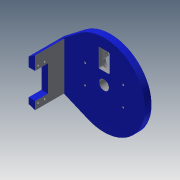
# Autodesk Inventor part: otocni_kruh(svrchni)
Saved by Autodesk Inventor 2013 (Build 170138000, 138)
## iProperties
Created: 2013-05-25
Part Number: otocni_kruh(svrchni)
Material: Generic
Document SubType Name: Modeling
Designer: idle-rug
Density: 1 g/cm^3
Author: idle-rug
Autodesk Inventor part; units mm, degrees
ref_plane "YZ Plane" through (0, 0, 0) normal (1, 0, 0) x (0, 1, 0)
ref_plane "XZ Plane" through (0, 0, 0) normal (0, 1, 0) x (-1, 0, 0)
ref_plane "XY Plane" through (0, 0, 0) normal (0, 0, 1) x (1, 0, 0)
sketch "Sketch1" plane through (0, 0, 0) normal (0, 1, 0) x (-1, 0, 0)
  circle A0 centre (0, 0) radius 60
  circle A1 centre (0, 0) radius 3
  dimension "d0" = 120
  dimension "d1" = 6
  constraints: 2 centre point, 2 coincident
  measures "d0" diameter of A0
  measures "d1" diameter of A1
extrude "Extrusion1" add sketch "Sketch1" along normal blind 10
sketch "Sketch2" plane through (0, 0, 0) normal (0, -1, 0) x (1, 0, 0)
  circle A0 centre (0, 0) radius 60 projected
  line L0 (0, 0) -> (24.3, 0)
  line L1 (24.3, 0) -> (29.3, 0)
  line L2 (0, 0) -> (-24.3, 0)
  line L3 (-24.3, 0) -> (-29.3, 0)
  line L4 (-24.3, 30) -> (-34.3, 30)
  line L5 (-34.3, 30) -> (-34.3, -30)
  line L6 (-34.3, -30) -> (-24.3, -30)
  line L7 (-24.3, -30) -> (-24.3, 30)
  line L8 (-24.3, 30) -> (-34.3, -30) construction
  line L9 (-34.3, 30) -> (-24.3, -30) construction
  line L10 (34.3, 30) -> (24.3, 30)
  line L11 (24.3, 30) -> (24.3, -30)
  line L12 (24.3, -30) -> (34.3, -30)
  line L13 (34.3, -30) -> (34.3, 30)
  line L14 (34.3, 30) -> (24.3, -30) construction
  line L15 (24.3, 30) -> (34.3, -30) construction
  line L16 (-29.3, 0) -> (-29.3, 15)
  line L17 (-29.3, 0) -> (-29.3, -15)
  line L18 (29.3, 0) -> (29.3, 15)
  line L19 (29.3, 0) -> (29.3, -15)
  circle A1 centre (29.3, -15) radius 1.5
  circle A2 centre (29.3, 15) radius 1.5
  circle A3 centre (-29.3, 15) radius 1.5
  circle A4 centre (-29.3, -15) radius 1.5
  dimension "d4" = 24.3
  dimension "d5" = 5
  dimension "d6" = 24.3
  dimension "d7" = 5
  dimension "d8" = 10
  dimension "d9" = 60
  dimension "d10" = 60
  dimension "d11" = 15
  dimension "d12" = 15
  dimension "d13" = 15
  dimension "d14" = 15
  dimension "d15" = 3
  dimension "d16" = 3
  dimension "d17" = 3
  dimension "d18" = 3
  constraints: 40 end point, 6 parallel, 5 collinear, 4 centre point, 4 coincident, 4 midpoint, 3 horizontal, 2 perpendicular
  measures "d4" distance of L0.start L0.end
  measures "d5" distance of L0.end L1.end
  measures "d6" distance of L0.start L2.end
  measures "d7" distance of L2.end L3.end
  measures "d8" distance of L6.end L5.end
  measures "d9" distance of L5.end L4.end
  measures "d10" distance of L11.end L10.end
  measures "d11" distance of L3.end L16.end
  measures "d12" distance of L3.end L17.end
  measures "d13" distance of L1.end L18.end
  measures "d14" distance of L1.end L19.end
  measures "d15" diameter of A1
  measures "d16" diameter of A2
  measures "d17" diameter of A3
  measures "d18" diameter of A4
extrude "Extrusion2" cut sketch "Sketch2" against normal blind 10 contours A1 | A2 | A3 | A4
sketch "Sketch3" plane through (0, 0, 0) normal (0, -1, 0) x (1, 0, 0)
  circle A0 centre (0, 0) radius 60 projected
  line L0 (0, 0) -> (-71.2, 0)
  line L1 (-71.2, 0) -> (-71.2, -34.25)
  line L2 (-71.2, -34.25) -> (-71.2, 20.75)
  line L3 (-24.1381, -54.9304) -> (-71.2, -34.25)
  line L4 (-36.7367, 47.4386) -> (-71.2, 20.75)
  arc A1 (-36.7367, 47.4386) -> (-24.1381, -54.9304) centre (0, 0) ccw
  dimension "d31" = 71.2
  dimension "d32" = 34.25
  dimension "d33" = 55
  constraints: 10 end point, 4 point on circle, 2 tangent, 1 centre point, 1 concentric, 1 horizontal, 1 perpendicular, 1 point on line
  measures "d31" distance of L0.start L0.end
  measures "d32" distance of L0.end L1.end
  measures "d33" distance of L1.end L2.end
extrude "Extrusion3" add sketch "Sketch3" against normal blind 10 contours A0 L0 L2 L4 | L3 L1 L0 A0
sketch "Sketch4" plane through (0, 0, 0) normal (0, -1, 0) x (1, 0, 0)
  line L0 (-61.2, 20.75) -> (-61.2, -34.25)
  line L1 (-71.2, -34.25) -> (-71.2, 20.75)
  line L2 (-61.2, 28.494) -> (-61.2, -38.6443)
  line L3 (-61.2, -38.6443) -> (-71.2, -34.25)
  line L4 (-71.2, -34.25) -> (-71.2, 20.75)
  line L5 (-71.2, -34.25) -> (-71.2, 20.75) projected
  line L6 (-61.2, 28.494) -> (-71.2, 20.75)
  dimension "d36" = 10
  constraints: 12 end point, 2 parallel, 1 collinear
  measures "d36" distance of L0.end L1.start
extrude "Extrusion4" add sketch "Sketch4" along normal blind 43
sketch "Sketch6" plane through (0, -43, 0) normal (0, -1, 0) x (1, 0, 0)
  line L0 (-71.2, 20.75) -> (-71.2, -34.25) projected
  line L1 (-71.2, -34.25) -> (-61.2, -38.6443) projected
  line L2 (-61.2, -38.6443) -> (-61.2, 28.494) projected
  line L3 (-61.2, 28.494) -> (-71.2, 20.75) projected
  point P0 (0, 0)
extrude "Extrusion5" add sketch "Sketch6" along normal blind 5
sketch "Sketch7" plane through (0, 10, 0) normal (0, 1, 0) x (1, 0, 0)
  arc A0 (-36.7367, -47.4386) -> (-24.1381, 54.9304) centre (0, 0) ccw projected
  line L0 (-24.1381, 54.9304) -> (-71.2, 34.25) projected
  line L1 (-71.2, 34.25) -> (-71.2, -20.75) projected
  line L2 (-71.2, -20.75) -> (-36.7367, -47.4386) projected
  line L3 (-71.2, 34.25) -> (-71.2, -20.75)
  line L4 (-71.2, -20.75) -> (-71.2, -24.75)
  line L5 (-71.2, 34.25) -> (-71.2, 38.25)
  line L6 (-71.2, 38.25) -> (-20.2127, 56.4929)
  line L7 (-71.2, -24.75) -> (-36.7367, -47.4386)
  line L8 (-71.2, -20.75) -> (-36.7367, -47.4386)
  line L9 (-71.2, 34.25) -> (-24.1381, 54.9304)
  arc A1 (-36.7367, -47.4386) -> (-24.1381, 54.9304) centre (0, 0) ccw projected
  arc A2 (-20.2127, 56.4929) -> (-24.1381, 54.9304) centre (0, 0) ccw
  dimension "d45" = 4
  dimension "d46" = 4
  constraints: 14 end point, 5 point on circle, 4 collinear, 2 point on line, 2 tangent, 1 centre point
  measures "d45" distance of L1.end L4.end
  measures "d46" distance of L0.end L5.end
extrude "Extrusion6" add sketch "Sketch7" against normal blind 10 contours L7 L4 L2 | A0 L0 L5 L6
sketch "Sketch8" plane through (0, 0, 0) normal (0, -1, 0) x (1, 0, 0)
  line L0 (-71.2, -38.25) -> (-20.2127, -56.4929) projected
  line L1 (-36.7367, 47.4386) -> (-71.2, 24.75) projected
  line L2 (-71.2, 24.75) -> (-71.2, 20.75) projected
  line L3 (-61.2, 28.494) -> (-71.2, 20.75) projected
  line L4 (-61.2, 28.494) -> (-61.2, 31.3334)
  line L5 (-61.2, -38.6443) -> (-61.2, -41.8279)
  line L6 (-71.2, -34.25) -> (-71.2, -38.25)
  line L7 (-71.2, -38.25) -> (-61.2, -41.8279)
  line L8 (-71.2, -34.25) -> (-61.2, -38.6443)
  line L9 (-71.2, -34.25) -> (-61.2, -38.6443) projected
  line L10 (-71.2, 20.75) -> (-71.2, 24.75)
  line L11 (-71.2, 24.75) -> (-61.2, 31.3334)
  line L12 (-61.2, 28.494) -> (-71.2, 20.75)
  constraints: 16 end point, 6 collinear, 2 parallel, 1 point on line
extrude "Extrusion7" add sketch "Sketch8" along normal blind 48
sketch "Sketch9" plane through (-71.2, -48, -38.25) normal (-1, 0, 0) x (0, 0, 1)
  line L0 (63, 58) -> (63, 0) projected
  line L1 (38.25, 48) -> (38.25, 13)
  line L2 (38.25, 13) -> (4, 13)
  line L3 (4, 13) -> (53.7, 13)
  line L4 (48.95, 23) -> (8.75, 23)
  line L5 (8.75, 23) -> (8.75, 3)
  line L6 (8.75, 3) -> (48.95, 3)
  line L7 (48.95, 3) -> (48.95, 23)
  line L8 (48.95, 23) -> (8.75, 3) construction
  line L9 (8.75, 23) -> (48.95, 3) construction
  circle A0 centre (53.7, 17.95) radius 1.5
  circle A1 centre (53.7, 8.05) radius 1.5
  circle A2 centre (4, 17.95) radius 1.5
  circle A3 centre (4, 8.05) radius 1.5
  point P0 (28.85, 13)
  dimension "d51" = 35
  dimension "d54" = 34.25
  dimension "d55" = 49.7
  dimension "d56" = 40.2
  dimension "d60" = 3
  dimension "d61" = 3
  dimension "d62" = 3
  dimension "d63" = 3
  constraints: 18 end point, 4 centre point, 3 midpoint, 3 parallel, 2 perpendicular, 1 horizontal, 1 point on line
  measures "d51" distance of L1.start L1.end
  measures "d54" distance of L1.end L2.end
  measures "d55" distance of L2.end L3.end
  measures "d56" distance of L6.end L5.end
  measures "d60" diameter of A0
  measures "d61" diameter of A1
  measures "d62" diameter of A2
  measures "d63" diameter of A3
extrude "Extrusion8" cut sketch "Sketch9" against normal blind 10
sketch "Sketch10" plane through (0, -48, 0) normal (0, -1, 0) x (1, 0, 0)
  line L0 (-71.2, 24.75) -> (-71.2, -38.25) projected
  line L1 (-71.2, -38.25) -> (-61.2, -41.8279) projected
  line L2 (-61.2, -41.8279) -> (-61.2, 31.3334) projected
  line L3 (-61.2, 31.3334) -> (-71.2, 24.75) projected
  point P0 (0, 0)
extrude "Extrusion9" cut sketch "Sketch10" against normal blind 3
sketch "Sketch11" plane through (0, 10, 0) normal (0, 1, 0) x (1, 0, 0)
  circle A0 centre (0, -37.2) radius 7.1045
  circle A1 centre (0, -37.2) radius 2
  dimension "d70" = 14.209
  dimension "d71" = 4
  constraints: 2 centre point, 1 coincident
  measures "d70" diameter of A0
  measures "d71" diameter of A1
extrude "Extrusion10" cut sketch "Sketch11" against normal blind 10 contours A1
sketch "Sketch12" plane through (0, 10, 0) normal (0, 1, 0) x (1, 0, 0)
  circle A0 centre (0, -37.2) radius 2 projected
  circle A1 centre (0, -37.2) radius 4
  dimension "d74" = 8
  constraints: 1 centre point, 1 coincident
  measures "d74" diameter of A1
extrude "Extrusion11" cut sketch "Sketch12" against normal blind 10
sketch "Sketch13" plane through (0, 0, 0) normal (0, -1, 0) x (1, 0, 0)
  circle A0 centre (0, 37.2) radius 4 projected
  circle A1 centre (0, 37.2) radius 4 projected
  circle A2 centre (0, 37.2) radius 7.5
  line L0 (0, 29.7) -> (0, 19.7)
  line L1 (0, 19.7) -> (-24.3, 19.7)
  line L2 (-24.3, 19.7) -> (-24.3, 54.859)
  line L3 (0, 19.7) -> (24.3, 19.7)
  line L4 (24.3, 19.7) -> (24.3, 54.859)
  arc A3 (24.3, 54.859) -> (-24.3, 54.859) centre (0, 0) ccw
  dimension "d78" = 15
  dimension "d79" = 10
  constraints: 10 end point, 2 perpendicular, 2 point on circle, 1 centre point, 1 coincident, 1 vertical alignment, 2 other
  measures "d79" distance of L0.start L0.end
extrude "Extrusion12" cut sketch "Sketch13" against normal blind 6 contours A2 | L1 L2 A3 L4 L3
sketch "Sketch14" plane through (0, 6, 0) normal (0, -1, 0) x (1, 0, 0)
  line L0 (-24.3, 19.7) -> (-24.3, 54.859) projected
  line L1 (24.3, 19.7) -> (-24.3, 19.7) projected
  line L2 (24.3, 54.859) -> (24.3, 19.7) projected
  arc A0 (24.3, 54.859) -> (-24.3, 54.859) centre (0, 0) ccw projected
  line L3 (-24.3, 19.7) -> (-10, 19.7)
  line L4 (-10, 19.7) -> (-10, 54.859)
  line L5 (-10, 54.859) -> (-24.3, 54.859)
  line L6 (-24.3, 54.859) -> (-24.3, 19.7)
  line L7 (24.3, 19.7) -> (10, 19.7)
  line L8 (10, 19.7) -> (10, 54.859)
  line L9 (10, 54.859) -> (24.3, 54.859)
  line L10 (24.3, 54.859) -> (24.3, 19.7)
  line L11 (-24.3, 54.859) -> (24.3, 54.859)
  dimension "d82" = 14.3
  dimension "d83" = 14.3
  constraints: 18 end point, 4 parallel, 2 horizontal, 2 perpendicular, 1 collinear
  measures "d82" distance of L5.end L4.end
  measures "d83" distance of L8.end L9.end
extrude "Extrusion13" add sketch "Sketch14" along normal blind 6 contours L0 L5 L4 L1 | A0 L9 L11 L5 | L2 L1 L8 L9
sketch "Sketch16" plane through (0, 0, 0) normal (0, -1, 0) x (1, 0, 0)
  line L0 (-10, 19.7) -> (-10, 29.7) projected
  line L1 (-10, 19.7) -> (-10, 54.859) projected
  line L2 (-10, 44.859) -> (-10, 54.859) projected
  line L3 (10, 54.859) -> (10, 44.859) projected
  line L4 (10, 54.859) -> (10, 19.7) projected
  line L5 (10, 29.7) -> (10, 19.7) projected
  arc A0 (-20.2127, -56.4929) -> (-36.7367, 47.4386) centre (0, 0) ccw projected
  circle A1 centre (0, 0) radius 3 projected
  circle A2 centre (0, 0) radius 24.3
  line L6 (-10, 54.859) -> (-24.3, 54.859)
  line L7 (-24.3, 54.859) -> (-24.3, 19.859)
  line L8 (-24.3, 19.859) -> (-10, 19.7)
  line L9 (10, 54.859) -> (24.3, 54.859)
  line L10 (24.3, 54.859) -> (24.3, 19.859)
  line L11 (24.3, 19.859) -> (10, 19.7)
  dimension "d90" = 48.6
  dimension "d91" = 14.3
  dimension "d92" = 35
  dimension "d93" = 14.3
  dimension "d94" = 35
  constraints: 12 end point, 2 perpendicular, 2 point on circle, 1 centre point, 1 coincident
  measures "d90" diameter of A2
  measures "d91" distance of L1.end L6.end
  measures "d92" distance of L6.end L7.end
  measures "d93" distance of L3.start L9.end
  measures "d94" distance of L9.end L10.end
extrude "Extrusion15" add sketch "Sketch16" along normal blind 24 contours L8 A2 L0 | A2 L8 L7 L6 L1 L0 | A2 L11 L4 | L4 L3 L9 L10 L11 A2
sketch "Sketch17" plane through (24.3, 0, 54.859) normal (1, 0, 0) x (0, 0, -1)
  line L0 (0, 0) -> (35, 0) projected
  line L1 (0, 0) -> (0, -24) projected
  line L2 (0, -24) -> (19.125, -24)
  line L3 (0, 0) -> (4.589, 0)
  line L4 (4.589, 0) -> (19.125, -24)
  line L5 (0, 0) -> (0, -24)
  point P0 (54.859, 0)
  dimension "d97" = 19.125
  dimension "d98" = 4.589
  constraints: 8 end point, 1 perpendicular, 1 point on line
  measures "d97" distance of L1.end L2.end
  measures "d98" distance of L0.start L3.end
extrude "Extrusion16" add sketch "Sketch17" along normal blind 10
sketch "Sketch18" plane through (-24.3, 0, 19.859) normal (-1, 0, 0) x (0, 0, 1)
  line L0 (0, 0) -> (35, 0) projected
  line L1 (35, 0) -> (35, -24) projected
  line L2 (35, -24) -> (15.875, -24)
  line L3 (35, -24) -> (-0.159, -24) projected
  line L4 (35, 0) -> (30.411, 0)
  line L5 (30.411, 0) -> (15.875, -24)
  point P0 (-19.859, 0)
  point P1 (25, -24)
  point P2 (9.841, -24)
  dimension "d101" = 19.125
  dimension "d102" = 4.589
  constraints: 6 end point, 2 point on line
  measures "d101" distance of L1.end L2.end
  measures "d102" distance of L0.end L4.end
extrude "Extrusion17" add sketch "Sketch18" along normal blind 10
sketch "Sketch23" plane through (0, 10, 0) normal (0, 1, 0) x (1, 0, 0)
  circle A0 centre (0, 0) radius 3 projected
  arc A1 (-36.7367, -47.4386) -> (-20.2127, 56.4929) centre (0, 0) ccw projected
  circle A2 centre (0, 0) radius 7.5
  dimension "d123" = 15
  constraints: 1 centre point, 1 coincident
  measures "d123" diameter of A2
extrude "Extrusion22" cut sketch "Sketch23" against normal blind 10
sketch "Sketch24" plane through (0, 0, 0) normal (0, -1, 0) x (1, 0, 0)
  arc A0 (-20.2127, -56.4929) -> (-36.7367, 47.4386) centre (0, 0) ccw projected
  circle A1 centre (0, 0) radius 17.5
  dimension "d126" = 35
  constraints: 1 centre point, 1 coincident
  measures "d126" diameter of A1
extrude "Extrusion23" add sketch "Sketch24" along normal blind 2
sketch "Sketch26" plane through (0, -2, 0) normal (0, -1, 0) x (1, 0, 0)
  circle A0 centre (0, 0) radius 17.5 projected
  circle A1 centre (0, 0) radius 5
  dimension "d131" = 10
  constraints: 1 centre point, 1 coincident
  measures "d131" diameter of A1
extrude "Extrusion24" cut sketch "Sketch26" against normal blind 2 contours A1
sketch "Sketch30" plane through (0, 10, 0) normal (0, 1, 0) x (1, 0, 0)
  arc A0 (-36.7367, -47.4386) -> (-20.2127, 56.4929) centre (0, 0) ccw projected
  line L0 (-20.2127, 56.4929) -> (-71.2, 38.25) projected
  line L1 (-71.2, 38.25) -> (-71.2, -24.75) projected
  line L2 (-71.2, -24.75) -> (-36.7367, -47.4386) projected
  line L3 (-71.2, 38.25) -> (-24.5824, 58.0061)
  line L4 (-71.2, -24.75) -> (-38.3769, -49.9621)
  line L5 (-71.2, 38.25) -> (-71.2, -24.75)
  line L6 (-71.2, 38.25) -> (-20.2127, 56.4929)
  line L7 (-71.2, -24.75) -> (-36.7367, -47.4386)
  arc A1 (-36.7367, -47.4386) -> (-20.2127, 56.4929) centre (0, 0) ccw
  arc A2 (-38.3769, -49.9621) -> (-24.5824, 58.0061) centre (0, 0) ccw
  dimension "d141" = 63
  constraints: 10 end point, 4 point on circle, 3 collinear, 2 centre point, 2 tangent, 1 concentric
  measures "d141" radius of A2
extrude "Extrusion27" add sketch "Sketch30" against normal blind 10 contours A0 L0 L3 A2 L4 L2
sketch "Sketch31" plane through (0, 10, 0) normal (0, 1, 0) x (1, 0, 0)
  circle A0 centre (0, -37.2) radius 4 projected
  line L0 (-71.2, 38.25) -> (-71.2, -24.75) projected
  line L1 (0, -33.2) -> (0, -25.7)
  circle A1 centre (0, -25.7) radius 7.5
  dimension "d144" = 7.5
  constraints: 2 end point, 2 vertical alignment, 1 coincident, 1 parallel, 3 other
  measures "d144" distance of L1.start L1.end
extrude "Extrusion28" cut sketch "Sketch31" against normal blind 10 contours A1
sketch "Sketch32" plane through (0, 10, 0) normal (0, 1, 0) x (1, 0, 0)
  line L0 (-71.2, 38.25) -> (-71.2, -24.75) projected
  circle A0 centre (0, -37.2) radius 4 projected
  circle A1 centre (0, -25.7) radius 7.5 projected
  line L1 (0, -33.2) -> (-3, -33.2)
  arc A2 (0, -33.2) -> (4.5, -19.7) centre (0, -25.7) ccw projected
  line L2 (-3, -33.2) -> (3, -33.2)
  line L3 (3, -32.2) -> (-3, -32.2)
  line L4 (-3, -32.2) -> (-3, -34.2)
  line L5 (-3, -34.2) -> (3, -34.2)
  line L6 (3, -34.2) -> (3, -32.2)
  line L7 (3, -32.2) -> (-3, -34.2) construction
  line L8 (-3, -32.2) -> (3, -34.2) construction
  line L9 (3, -31.8458) -> (-3, -31.8458)
  line L10 (-3, -31.8458) -> (-3, -34.5542)
  line L11 (-3, -34.5542) -> (3, -34.5542)
  line L12 (3, -34.5542) -> (3, -31.8458)
  line L13 (3, -31.8458) -> (-3, -34.5542) construction
  line L14 (-3, -31.8458) -> (3, -34.5542) construction
  point P0 (6.3443, -29.7)
  dimension "d147" = 3
  dimension "d148" = 6
  dimension "d149" = 2
  constraints: 28 end point, 4 midpoint, 4 parallel, 3 perpendicular, 3 tangent, 2 horizontal, 1 collinear, 1 point on circle
  measures "d147" distance of L1.start L1.end
  measures "d148" distance of L1.end L2.end
  measures "d149" distance of L5.end L3.start
extrude "Extrusion29" cut sketch "Sketch32" against normal blind 10 contours L11 A0 L5 | A0 L5 L12 | L10 L5 A0 | L5 A0 | A0 L2 L6 L5 | L5 L4 L1 A0 | L1 L4 A1 | A1 L4 L3 L6 | A1 L6 L2 | L10 L9 L12 L3
sketch "Sketch33" plane through (0, -24, 0) normal (0, -1, 0) x (1, 0, 0)
  line L0 (10, 19.7) -> (24.3, 19.859) projected
  line L1 (24.3, 19.859) -> (24.3, 35.734) projected
  line L2 (24.3, 35.734) -> (34.3, 35.734) projected
  line L3 (34.3, 54.859) -> (34.3, 35.734) projected
  line L4 (10, 54.859) -> (34.3, 54.859) projected
  line L5 (10, 54.859) -> (10, 19.7) projected
  point P0 (0, 0)
extrude "Extrusion30" cut sketch "Sketch33" against normal blind 24
sketch "Sketch34" plane through (0, -24, 0) normal (0, -1, 0) x (1, 0, 0)
  line L0 (-10, 19.7) -> (-10, 54.859) projected
  line L1 (-10, 54.859) -> (-34.3, 54.859) projected
  line L2 (-34.3, 35.734) -> (-34.3, 54.859) projected
  line L3 (-24.3, 35.734) -> (-34.3, 35.734) projected
  line L4 (-24.3, 35.734) -> (-24.3, 19.859) projected
  line L5 (-24.3, 19.859) -> (-10, 19.7) projected
  point P0 (0, 0)
extrude "Extrusion31" cut sketch "Sketch34" against normal blind 24
sketch "Sketch35" plane through (0, 0, 0) normal (0, -1, 0) x (1, 0, 0)
  arc A0 (-4.5, 19.7) -> (4.5, 19.7) centre (0, 25.7) ccw projected
  line L0 (-61.2, 31.3334) -> (-61.2, -41.8279) projected
  line L1 (0, 18.2) -> (-10, 18.2)
  line L2 (-10, 19.7) -> (-10, 18.2)
  line L3 (-10, 19.7) -> (10, 19.7)
  line L4 (10, 19.7) -> (10, 18.2)
  line L5 (10, 18.2) -> (-10, 18.2)
  line L6 (-10, 18.2) -> (-10, 19.7)
  constraints: 12 end point, 3 perpendicular, 2 parallel, 1 horizontal, 1 point on circle, 1 tangent
extrude "Extrusion32" cut sketch "Sketch35" against normal blind 6
sketch "Sketch36" plane through (0, 6, 0) normal (0, -1, 0) x (1, 0, 0)
  arc A0 (3, 34.5542) -> (-3, 34.5542) centre (0, 37.2) ccw projected
  line L0 (10, 18.2) -> (10, 54.859) projected
  line L1 (10, 54.859) -> (-10, 54.859) projected
  line L2 (-10, 54.859) -> (-10, 18.2) projected
  line L3 (7.5, 49.2) -> (-7.5, 49.2)
  line L4 (-7.5, 49.2) -> (-7.5, 25.2)
  line L5 (-7.5, 25.2) -> (7.5, 25.2)
  line L6 (7.5, 25.2) -> (7.5, 49.2)
  line L7 (7.5, 49.2) -> (-7.5, 25.2) construction
  line L8 (-7.5, 49.2) -> (7.5, 25.2) construction
  line L9 (-10, 49.2) -> (10, 49.2)
  point P0 (0, 0)
  dimension "d158" = 15
  dimension "d159" = 24
  constraints: 14 end point, 3 point on line, 2 midpoint, 2 parallel, 1 horizontal, 1 perpendicular
  measures "d158" distance of L5.end L4.end
  measures "d159" distance of L4.end L3.end
extrude "Extrusion33" add sketch "Sketch36" along normal blind 6 contours L9 L3 L2 L1 L0
sketch "Sketch37" plane through (0, 6, 0) normal (0, -1, 0) x (1, 0, 0)
  line L0 (10, 49.2) -> (-10, 49.2) projected
  line L1 (-10, 49.2) -> (-10, 18.2) projected
  line L2 (10, 18.2) -> (10, 49.2) projected
  line L3 (8, 47.2) -> (-8, 47.2)
  line L4 (-8, 47.2) -> (-8, 27.2)
  line L5 (-8, 27.2) -> (8, 27.2)
  line L6 (8, 27.2) -> (8, 47.2)
  arc A0 (3, 34.5542) -> (-3, 34.5542) centre (0, 37.2) ccw projected
  line L7 (8, 47.2) -> (-8, 27.2) construction
  line L8 (-8, 47.2) -> (8, 27.2) construction
  line L9 (-10, 47.2) -> (10, 47.2)
  point P0 (0, 0)
  dimension "d162" = 16
  dimension "d163" = 20
  constraints: 14 end point, 2 midpoint, 2 parallel, 2 perpendicular, 2 point on line, 1 horizontal
  measures "d162" distance of L5.end L4.end
  measures "d163" distance of L4.end L3.end
extrude "Extrusion34" add sketch "Sketch37" along normal blind 6 contours L2 L9 L3 L1 L0
sketch "Sketch38" plane through (0, 6, 0) normal (0, -1, 0) x (1, 0, 0)
  line L0 (-10, 47.2) -> (-10, 18.2) projected
  line L1 (0, 18.2) -> (-10, 18.2) projected
  arc A0 (3, 34.5542) -> (-3, 34.5542) centre (0, 37.2) ccw projected
  line L2 (10, 18.2) -> (0, 18.2) projected
  line L3 (10, 18.2) -> (10, 47.2) projected
  line L4 (-10, 47.2) -> (10, 47.2) projected
  line L5 (8.5, 27.2) -> (-8.5, 27.2)
  line L6 (-8.5, 27.2) -> (-8.5, 47.2)
  line L7 (-8.5, 47.2) -> (8.5, 47.2)
  line L8 (8.5, 47.2) -> (8.5, 27.2)
  line L9 (8.5, 27.2) -> (-8.5, 47.2) construction
  line L10 (-8.5, 27.2) -> (8.5, 47.2) construction
  line L11 (-8.5, 47.2) -> (-8.5, 18.2)
  line L12 (8.5, 47.2) -> (8.5, 18.2)
  line L13 (10, 18.2) -> (-10, 18.2) projected
  point P0 (0, 0)
  dimension "d166" = 17
  constraints: 16 end point, 3 parallel, 3 point on line, 2 midpoint, 2 perpendicular, 1 horizontal
  measures "d166" distance of L6.end L7.end
extrude "Extrusion35" add sketch "Sketch38" along normal blind 6 contours L4 L6 L11 L1 L0 | L4 L3 L2 L12 L8
fillet "Fillet9" radius 2 4 edges at (8.5, 3, 18.2) (-8.5, 3, 18.2) (-8.5, 3, 47.2) (8.5, 3, 47.2)
sketch "Sketch39" plane through (0, -2, 0) normal (0, -1, 0) x (1, 0, 0)
  circle A0 centre (0, 0) radius 5 projected
  circle A1 centre (0, 0) radius 17.5 projected
extrude "Extrusion36" cut sketch "Sketch39" against normal blind 2
body "Solid1"
